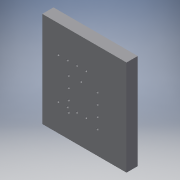
# Autodesk Inventor part: Trasera
Saved by Autodesk Inventor 2017 (Build 210142000, 142)
## iProperties
Created: 2021-02-12
Part Number: Trasera
Material: Generic
Document SubType Name: Modeling
Designer: USUARIO
Density: 1 g/cm^3
Appearance: Default
Author: USUARIO
Autodesk Inventor part; units mm, degrees
ref_plane "YZ Plane" through (0, 0, 0) normal (1, 0, 0) x (0, 1, 0)
ref_plane "XZ Plane" through (0, 0, 0) normal (0, 1, 0) x (-1, 0, 0)
ref_plane "XY Plane" through (0, 0, 0) normal (0, 0, 1) x (1, 0, 0)
sketch "Sketch1" plane through (0, 0, 0) normal (0, 1, 0) x (-1, 0, 0)
  line L0 (0, 0) -> (380, 0)
  line L1 (380, 0) -> (380, -430)
  line L2 (380, -430) -> (0, -430)
  line L3 (0, -430) -> (0, 0)
  dimension "d0" = 380
  dimension "d1" = 430
  constraints: 8 end point, 2 parallel, 1 horizontal, 1 perpendicular
  measures "d0" distance of L1.end L2.end
  measures "d1" distance of L0.end L1.end
extrude "Extrusion1" add sketch "Sketch1" along normal blind 50.8
sketch "Sketch2" plane through (0, 50.8, 0) normal (0, 1, 0) x (1, 0, 0)
  circle A0 centre (-220, 215) radius 5
  line L0 (0, 430) -> (-380, 430) projected
  line L1 (0, 0) -> (0, 430) projected
  line L2 (-380, 430) -> (-380, 0) projected
  dimension "d4" = 10
  dimension "d10" = 215
  dimension "d11" = 160
  constraints: 1 centre point
  measures "d4" diameter of A0
  measures "d10" distance from line of L0 A0.centre
  measures "d11" distance from line of L2 A0.centre
extrude "Extrusion2" cut sketch "Sketch2" against normal blind 50.8
sketch "Sketch3" plane through (0, 50.8, 0) normal (0, 1, 0) x (1, 0, 0)
  circle A0 centre (-170, 130) radius 5
  line L0 (0, 0) -> (0, 430) projected
  line L1 (-380, 0) -> (0, 0) projected
  circle A1 centre (-190, 130) radius 5
  circle A2 centre (-210, 130) radius 5
  circle A3 centre (-230, 130) radius 5
  dimension "d12" = 10
  dimension "d13" = 170
  dimension "d14" = 130
  dimension "d20" = 20
  constraints: 4 centre point, 1 horizontal, 6 other
  measures "d12" diameter of A0
  measures "d13" distance from line of A0.centre L0
  measures "d14" distance from line of A0.centre L1
  measures "d20" distance of A0.centre A1.centre
extrude "Extrusion3" cut sketch "Sketch3" against normal blind 50.8
sketch "Sketch4" plane through (0, 50.8, 0) normal (0, 1, 0) x (1, 0, 0)
  circle A0 centre (-170, 300) radius 5
  line L0 (0, 0) -> (0, 430) projected
  line L1 (0, 430) -> (-380, 430) projected
  circle A1 centre (-190, 300) radius 5
  circle A2 centre (-210, 300) radius 5
  circle A3 centre (-230, 300) radius 5
  dimension "d24" = 10
  dimension "d25" = 170
  dimension "d26" = 130
  dimension "d32" = 20
  constraints: 4 centre point, 1 horizontal, 6 other
  measures "d24" diameter of A0
  measures "d25" distance from line of A0.centre L0
  measures "d26" distance from line of A0.centre L1
  measures "d32" distance of A0.centre A1.centre
extrude "Extrusion4" cut sketch "Sketch4" against normal blind 50.8
sketch "Sketch5" plane through (0, 50.8, 0) normal (0, 1, 0) x (1, 0, 0)
  circle A0 centre (-260, 170) radius 5
  line L0 (-380, 430) -> (-380, 0) projected
  line L1 (-380, 0) -> (0, 0) projected
  circle A1 centre (-140, 170) radius 5
  line L2 (0, 0) -> (0, 430) projected
  circle A2 centre (-260, 200) radius 5
  circle A3 centre (-140, 200) radius 5
  circle A4 centre (-260, 230) radius 5
  circle A5 centre (-140, 230) radius 5
  circle A6 centre (-260, 260) radius 5
  circle A7 centre (-140, 260) radius 5
  dimension "d36" = 10
  dimension "d37" = 120
  dimension "d38" = 170
  dimension "d39" = 10
  dimension "d40" = 170
  dimension "d41" = 140
  dimension "d47" = 30
  constraints: 8 centre point, 1 vertical, 12 other
  measures "d36" diameter of A0
  measures "d37" distance from line of A0.centre L0
  measures "d38" distance from line of A0.centre L1
  measures "d39" diameter of A1
  measures "d40" distance from line of A1.centre L1
  measures "d41" distance from line of A1.centre L2
  measures "d47" distance of A0.centre A2.centre
extrude "Extrusion5" cut sketch "Sketch5" against normal blind 50.8
body "Solid1"
